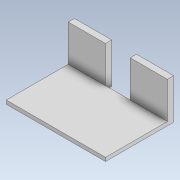
# Autodesk Inventor part: electrical_system_fix_board
Saved by Autodesk Inventor 2020 (Build 240168000, 168)
## iProperties
Created: 2021-01-08
Part Number: electrical_system_fix_board
Material: Generic
Document SubType Name: Modeling
Designer: DELL
Density: 1 g/cm^3
Appearance: Default
Author: DELL
Autodesk Inventor part; units mm, degrees
ref_plane "YZ Plane" through (0, 0, 0) normal (1, 0, 0) x (0, 1, 0)
ref_plane "XZ Plane" through (0, 0, 0) normal (0, 1, 0) x (-1, 0, 0)
ref_plane "XY Plane" through (0, 0, 0) normal (0, 0, 1) x (1, 0, 0)
sketch "Sketch1" plane through (0, 0, 0) normal (0, 0, 1) x (1, 0, 0)
  line L0 (80, 32.5) -> (-80, 32.5)
  line L1 (-80, 32.5) -> (-80, -32.5)
  line L2 (-80, -32.5) -> (80, -32.5)
  line L3 (80, -32.5) -> (80, 32.5)
  line L4 (80, 32.5) -> (-80, -32.5) construction
  line L5 (-80, 32.5) -> (80, -32.5) construction
  line L6 (-20, -32.5) -> (-80, -32.5)
  line L7 (-80, -32.5) -> (-80, 32.5)
  line L8 (-80, 32.5) -> (-20, 32.5)
  line L9 (-20, 32.5) -> (-20, -32.5)
  line L10 (-20, -32.5) -> (-80, 32.5) construction
  line L11 (-80, -32.5) -> (-20, 32.5) construction
  line L12 (20, -32.5) -> (80, -32.5)
  line L13 (80, -32.5) -> (80, 32.5)
  line L14 (80, 32.5) -> (20, 32.5)
  line L15 (20, 32.5) -> (20, -32.5)
  line L16 (20, -32.5) -> (80, 32.5) construction
  line L17 (80, -32.5) -> (20, 32.5) construction
  line L18 (0, 32.5) -> (0, -32.5) construction
  point P0 (0, 0)
  point P1 (-50, 0)
  point P2 (50, 0)
  point P3 (20, 32.5)
  point P4 (20, -32.5)
  point P5 (-20, -32.5)
  point P6 (-20, 32.5)
  dimension "d0" = 160
  dimension "d1" = 65
  dimension "d2" = 40
  constraints: 38 end point, 8 midpoint, 6 parallel, 3 horizontal, 3 perpendicular, 2 collinear, 1 other
  measures "d0" distance between parallel lines of L3 L1
  measures "d1" distance between parallel lines of L2 L0
  measures "d2" distance between parallel lines of L15 L9
extrude "Extrusion1" add sketch "Sketch1" along normal blind 10 contours L3 L2 L15 L0 | L9 L2 L1 L0
sketch "Sketch2" plane through (0, 0, 10) normal (0, 0, 1) x (1, 0, 0)
  line L0 (-80, -32.5) -> (-20, -32.5) projected
  line L1 (80, -26.5) -> (-80, -26.5)
  line L2 (-80, -26.5) -> (-80, -32.5)
  line L3 (-80, -32.5) -> (80, -32.5)
  line L4 (80, -32.5) -> (80, -26.5)
  line L5 (80, -26.5) -> (-80, -32.5) construction
  line L6 (-80, -26.5) -> (80, -32.5) construction
  line L7 (80, -32.5) -> (80, 32.5) projected
  point P0 (0, 0)
  point P1 (0, -29.5)
  dimension "d5" = 6
  constraints: 12 end point, 2 midpoint, 2 parallel, 1 collinear, 1 horizontal, 1 perpendicular
  measures "d5" distance between parallel lines of L3 L1
extrude "Extrusion2" add sketch "Sketch2" along normal blind 100
body "Solid1"
